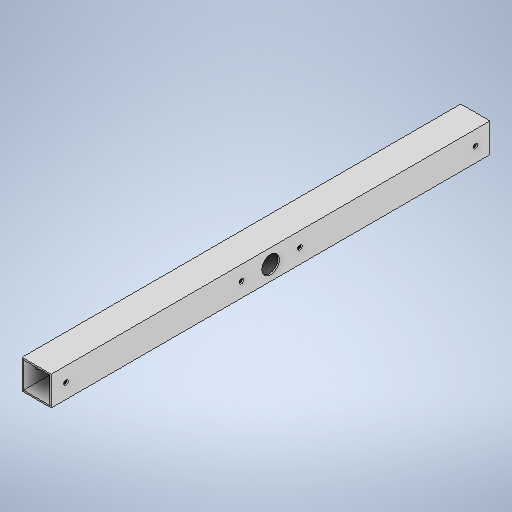
# Autodesk Inventor part: xx_shita
Saved by Autodesk Inventor 2025.1 (Build 291241000, 241)
## iProperties
Created: 2024-12-04
Part Number: xx_shita
Material: 一般
Document SubType Name: Modeling
Designer: yuki0520
Density: 1 g/cm^3
Appearance: 既定
Author: yuki0520
Autodesk Inventor part; units mm, degrees
ref_plane "YZ Plane" through (0, 0, 0) normal (1, 0, 0) x (0, 1, 0)
ref_plane "XZ Plane" through (0, 0, 0) normal (0, 1, 0) x (-1, 0, 0)
ref_plane "XY Plane" through (0, 0, 0) normal (0, 0, 1) x (1, 0, 0)
sketch "スケッチ1" plane through (0, 0, 0) normal (0, 0, 1) x (1, 0, 0)
  line L0 (10, -10) -> (-10, -10)
  line L1 (-10, -10) -> (-10, 10)
  line L2 (-10, 10) -> (10, 10)
  line L3 (10, 10) -> (10, -10)
  line L4 (10, -10) -> (-10, 10) construction
  line L5 (-10, -10) -> (10, 10) construction
  line L6 (9, 9) -> (-9, 9)
  line L7 (-9, 9) -> (-9, -9)
  line L8 (-9, -9) -> (9, -9)
  line L9 (9, -9) -> (9, 9)
  point P0 (0, 0)
  dimension "d0" = 20
  dimension "d1" = 20
  dimension "d2" = 1
  constraints: 20 end point, 4 parallel, 2 midpoint, 2 perpendicular, 1 horizontal, 3 other
  measures "d0" distance of L1.end L2.end
  measures "d1" distance of L0.end L1.end
  measures "d2" distance between parallel lines of L2 L6
extrude "押し出し1" add sketch "スケッチ1" along normal blind 300
sketch "スケッチ2" plane through (10, -10, 0) normal (1, 0, 0) x (0, 0, -1)
  line L0 (0, 10) -> (-300, 10)
  line L1 (-300, 0) -> (-300, 20) projected
  line L2 (0, 0) -> (0, 20) projected
  point P0 (-290, 10)
  point P1 (-10, 10)
  point P2 (-150, 10)
  point P3 (-170, 10)
  point P4 (-130, 10)
  dimension "d5" = 10
  dimension "d6" = 10
  dimension "d17" = 20
  dimension "d18" = 20
  constraints: 4 point on line, 2 end point, 2 midpoint
  measures "d5" distance from line of L1 point (-290, 10)
  measures "d6" distance from line of L2 point (-10, 10)
  measures "d17" distance of point (-170, 10) point (-150, 10)
  measures "d18" distance of point (-130, 10) point (-150, 10)
hole "穴1" at (10, 0, 290) at (10, 0, 10) at (10, 0, 170) at (10, 0, 130) direction (-1, 0, 0) diameter 3.2 end through all
sketch "スケッチ3" plane through (10, -10, 0) normal (1, 0, 0) x (0, 0, -1)
  line L0 (0, 10) -> (-300, 10)
  line L1 (-300, 1) -> (-300, 19) projected
  circle A0 centre (-150, 10) radius 6
  dimension "d14" = 12
  constraints: 2 end point, 2 midpoint, 1 centre point
  measures "d14" diameter of A0
extrude "押し出し2" cut sketch "スケッチ3" against normal blind 300
